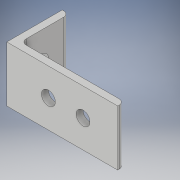
# Autodesk Inventor part: L bracket
Saved by Autodesk Inventor 2017 (Build 210142000, 142)
## iProperties
Created: 2016-09-29
Part Number: L bracket
Material: Generic
Document SubType Name: Modeling
Designer: Hanson
Density: 1 g/cm^3
Appearance: Default
Author: Hanson
Autodesk Inventor part; units mm, degrees
ref_plane "YZ Plane" through (0, 0, 0) normal (1, 0, 0) x (0, 1, 0)
ref_plane "XZ Plane" through (0, 0, 0) normal (0, 1, 0) x (-1, 0, 0)
ref_plane "XY Plane" through (0, 0, 0) normal (0, 0, 1) x (1, 0, 0)
sketch "Sketch1" plane through (0, 0, 0) normal (1, 0, 0) x (0, 1, 0)
  line L0 (0, 0) -> (-25.4, 0)
  line L1 (-25.4, 0) -> (-25.4, -25.4)
  line L2 (-25.4, -25.4) -> (0, -25.4)
  line L3 (0, -25.4) -> (0, 0)
  dimension "d0" = 25.4
  dimension "d1" = 25.4
  constraints: 8 end point, 2 parallel, 1 horizontal, 1 perpendicular
  measures "d0" distance of L2.end L1.end
  measures "d1" distance of L1.end L0.end
extrude "Extrusion1" add sketch "Sketch1" along normal blind 3.175
sketch "Sketch2" plane through (3.175, 0, 0) normal (1, 0, 0) x (0, 0, -1)
  line L0 (0, 0) -> (3.175, 0)
  line L1 (3.175, 0) -> (3.175, -25.4)
  line L2 (3.175, -25.4) -> (0, -25.4)
  line L3 (0, -25.4) -> (0, 0)
  dimension "d4" = 3.175
  dimension "d5" = 25.4
  constraints: 8 end point, 2 parallel, 1 horizontal, 1 perpendicular
  measures "d4" distance of L1.end L2.end
  measures "d5" distance of L0.end L1.end
extrude "Extrusion2" add sketch "Sketch2" along normal blind 47.625
sketch "Sketch3" plane through (3.175, -25.4, -3.175) normal (0, 0, -1) x (-1, 0, 0)
  line L0 (-47.625, 0) -> (-47.625, 25.4) projected
  line L1 (0, 0) -> (0, 25.4) projected
  line L2 (0, 0) -> (-47.625, 0) projected
  point P0 (3.175, 25.4)
  point P1 (-31.75, 12.7)
  point P2 (-15.875, 12.7)
  dimension "d8" = 15.875
  dimension "d9" = 15.875
  dimension "d10" = 15.875
  dimension "d11" = 12.7
  measures "d8" distance from line of L0 point (-31.75, 12.7)
  measures "d9" distance of point (-31.75, 12.7) point (-15.875, 12.7)
  measures "d10" distance from line of L1 point (-15.875, 12.7)
  measures "d11" distance from line of L2 point (-15.875, 12.7)
hole "Hole1" at (34.925, -12.7, -3.175) at (19.05, -12.7, -3.175) direction (0, 0, 1) diameter 6.35 end through all
sketch "Sketch4" plane through (3.175, 0, 0) normal (1, 0, 0) x (0, 0, -1)
  line L0 (25.4, 0) -> (3.175, 0) projected
  line L1 (25.4, -25.4) -> (25.4, 0) projected
  point P0 (0, 0)
  point P1 (12.7, -12.7)
  dimension "d19" = 12.7
  dimension "d20" = 12.7
  measures "d19" distance from line of L0 point (12.7, -12.7)
  measures "d20" distance from line of L1 point (12.7, -12.7)
hole "Hole2" at (3.175, -12.7, -12.7) direction (-1, 0, 0) diameter 6.35 end through all
fillet "Fillet1" radius 2.54 1 edges at (50.8, -12.7, -3.175)
fillet "Fillet2" radius 2.54 1 edges at (3.175, -12.7, -3.175)
fillet "Fillet3" radius 2.54 1 edges at (3.175, -12.7, -25.4)
body "Solid1"
